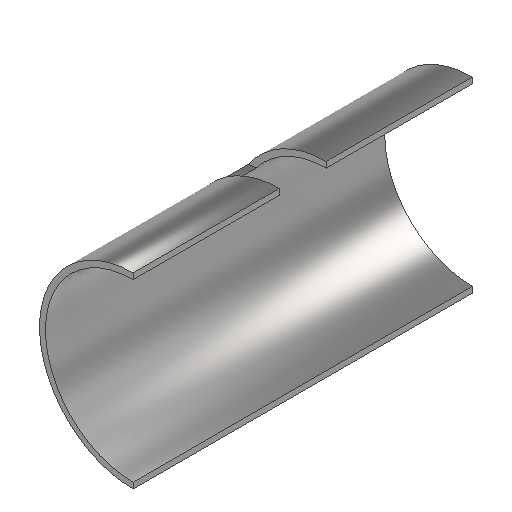
# Autodesk Inventor part: cover-pipe_L58
Saved by Autodesk Inventor 2026.2 (Build 302298000, 298)
## iProperties
Created: 2025-10-23
Part Number: cover-pipe_L58
Material: ステンレス鋼
Document SubType Name: Modeling
Designer: jin20
Density: 8 g/cm^3
Appearance: 半つや出し
Author: jin20
Autodesk Inventor part; units mm, degrees
ref_plane "YZ Plane" through (0, 0, 0) normal (1, 0, 0) x (0, 1, 0)
ref_plane "XZ Plane" through (0, 0, 0) normal (0, 1, 0) x (-1, 0, 0)
ref_plane "XY Plane" through (0, 0, 0) normal (0, 0, 1) x (1, 0, 0)
sketch "スケッチ1" plane through (0, 0, 0) normal (1, 0, 0) x (0, 1, 0)
  line L0 (0, 0) -> (15, 0) construction
  line L1 (15, 0) -> (15, -48) construction
  line L2 (15, -48) -> (16, -48)
  line L3 (16, -48) -> (16, 10)
  line L4 (16, 10) -> (15, 10)
  line L5 (15, 10) -> (15, -48)
  line L6 (0, -59.6) -> (0, 21.6) projected
  dimension "d0" = 15
  dimension "d2" = 1
  dimension "d3" = 58
  constraints: 12 end point, 2 horizontal, 2 parallel, 2 perpendicular
  measures "d0" distance of L0.start L0.end
  measures "d2" distance of L4.end L3.end
  measures "d3" distance of L3.end L2.end
revolve "回転1" add sketch "スケッチ1" angle 180 about axis through (0, 0, -10) along (0, 0, 1)
sketch "スケッチ2" plane through (0, 15, 10) normal (1, 0, 0) x (0, 0, -1)
  line L0 (58, 1) -> (0, 1) projected
  line L1 (0, 1) -> (25, 1)
  line L2 (25, 1) -> (33, 1)
  line L3 (33, 1) -> (33, -6)
  line L4 (33, -6) -> (25, -6)
  line L5 (25, -6) -> (25, 1)
  line L6 (0, 1) -> (0, 0) projected
  point P0 (10, -15)
  point P1 (33, 1)
  dimension "d6" = 8
  dimension "d7" = 7
  dimension "d10" = 25
  constraints: 10 end point, 2 parallel, 1 horizontal, 1 perpendicular, 1 point on line
  measures "d6" distance of L3.end L4.end
  measures "d7" distance of L2.end L3.end
  measures "d10" distance between parallel lines of L5 L6
extrude "押し出し1" cut sketch "スケッチ2" against normal through all
